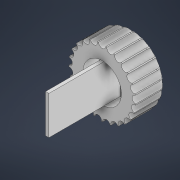
# Autodesk Inventor part: Turn knob
Saved by Autodesk Inventor 2021 (Build 250183000, 183)
## iProperties
Created: 2021-06-29
Part Number: Turn knob
Material: Generic
Document SubType Name: Modeling
Designer: allen
Density: 1 g/cm^3
Appearance: Default
Author: allen
Autodesk Inventor part; units mm, degrees
ref_plane "YZ Plane" through (0, 0, 0) normal (1, 0, 0) x (0, 1, 0)
ref_plane "XZ Plane" through (0, 0, 0) normal (0, 1, 0) x (-1, 0, 0)
sketch "Sketch1" plane through (0, 0, 0) normal (1, 0, 0) x (0, 1, 0)
  line L0 (0, -24.8075) -> (0, 4.1346) projected
  line L1 (0, 0) -> (5.5, 0)
  line L2 (5.5, 0) -> (5.5, -5)
  line L3 (5.5, -5) -> (0, -5)
  line L4 (0, -5) -> (0, 0)
  line L5 (3.15, 0) -> (3.15, -5)
  dimension "d0" = 11
  dimension "d1" = 5
  dimension "d2" = 6.3
  constraints: 10 end point, 2 parallel, 2 point on line, 1 horizontal, 1 perpendicular, 1 vertical
  measures "d0" diameter of L2 L0
  measures "d1" distance of L1.end L2.end
  measures "d2" diameter of L5 L0
revolve "Revolution1" add sketch "Sketch1" angle 360 about axis through (0, 0, -10) along (0, 0, 1) contours L5 L1 L2 L3
sketch "Sketch2" plane through (0, 0, -5) normal (0, 0, -1) x (-1, 0, 0)
  circle A0 centre (0, 0) radius 5.5 projected
extrude "Extrusion1" add sketch "Sketch2" against normal blind 2.35
sketch "Sketch3" plane through (0, 0, -2.65) normal (0, 0, 1) x (1, 0, 0)
  circle A0 centre (0, 0) radius 3.15 construction
  circle A1 centre (0, 0) radius 3.15 construction
  line L0 (0.275, -3.138) -> (0.275, 3.138)
  line L1 (-0.275, -3.138) -> (-0.275, 3.138)
  line L2 (0.275, 0) -> (-0.275, 0) construction
  arc A2 (-0.275, -3.138) -> (0.275, -3.138) centre (0, 0) ccw
  arc A3 (0.275, 3.138) -> (-0.275, 3.138) centre (0, 0) ccw
  dimension "d1" = 5
  dimension "d7" = 0.55
  constraints: 8 point on circle, 6 end point, 3 midpoint, 2 centre point, 2 concentric, 2 vertical, 1 coincident, 1 perpendicular
  measures "d7" distance between parallel lines of L1 L0
ref_plane "Work Plane1" through (0, 0, 9) normal (0, 0, -1) x (-1, 0, 0)
sketch "Sketch4" plane through (0, 0, 9) normal (0, 0, -1) x (-1, 0, 0)
  line L0 (-0.275, -3.138) -> (-0.275, 3.138) projected
  line L1 (0.275, -3.138) -> (0.275, 3.138) projected
  arc A0 (0.275, -3.138) -> (0.275, 3.138) centre (0, 0) ccw construction
  arc A1 (-0.275, -3.138) -> (0.275, -3.138) centre (0, 0) ccw
  arc A2 (0.275, 3.138) -> (-0.275, 3.138) centre (0, 0) ccw
  arc A3 (-0.275, 3.138) -> (-0.275, -3.138) centre (0, 0) ccw construction
  constraints: 8 point on circle, 4 centre point, 4 end point, 1 coincident
loft "Loft1" add profiles "Sketch3", "Sketch4"
sketch "Sketch5" plane through (0, 0, -5) normal (0, 0, -1) x (-1, 0, 0)
  circle A0 centre (0, 0) radius 5.5 projected
  arc A1 (-0.5991, 5.4673) -> (0.5991, 5.4673) centre (0, 5.5) ccw
  point P0 (0, 4.9)
  dimension "d13" = 0.6
  constraints: 6 point on circle, 1 centre point, 1 vertical alignment
  measures "d13" radius of A1
fillet "Fillet1" radius 1 1 edges at (0, -5.5, -5)
extrude "Extrusion2" cut sketch "Sketch5" against normal through all contours A1 A0 picked at (-0.0233, 5.2989)
pattern_circular "Circular Pattern1" count 25 over 360 about axis through (0, 0, -2.5) along (0, 0, -1) of "Extrusion2"
body "Solid1"
